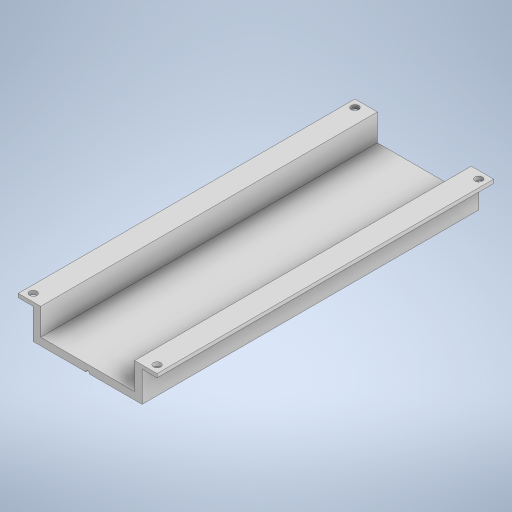
# Autodesk Inventor part: SoporteMaterial
Saved by Autodesk Inventor 2023 (Build 270158000, 158)
## iProperties
Created: 2023-04-09
Part Number: SoporteMaterial
Material: Generic
Document SubType Name: Modeling
Designer: Lenovo
Density: 1 g/cm^3
Appearance: Default
Author: Lenovo
Autodesk Inventor part; units mm, degrees
ref_plane "YZ Plane" through (0, 0, 0) normal (1, 0, 0) x (0, 1, 0)
ref_plane "XZ Plane" through (0, 0, 0) normal (0, 1, 0) x (-1, 0, 0)
ref_plane "XY Plane" through (0, 0, 0) normal (0, 0, 1) x (1, 0, 0)
sketch "Sketch1" plane through (0, 0, 0) normal (0, 0, 1) x (1, 0, 0)
  line L0 (165.5, 18.25) -> (165.5, 13.25)
  line L1 (95.5, -27.5) -> (75.25, -27.5)
  arc A0 (75.25, -27.5) -> (70.25, -27.5) centre (72.75, -27.5) ccw
  line L2 (70.25, -27.5) -> (50, -27.5)
  line L3 (145.5, 0) -> (145.5, 13.25)
  line L4 (145.5, 13.25) -> (165.5, 13.25)
  line L5 (0, 13.25) -> (0, 0)
  line L6 (0, 13.25) -> (-20, 13.25)
  line L7 (-20, 13.25) -> (-20, 18.25)
  line L8 (-20, 18.25) -> (0, 18.25)
  line L9 (0, 18.25) -> (10, 18.25)
  line L10 (10, 18.25) -> (10, -17.5)
  line L11 (165.5, 18.25) -> (145.5, 18.25)
  line L12 (145.5, 18.25) -> (135.5, 18.25)
  line L13 (135.5, 18.25) -> (135.5, -17.5)
  line L14 (135.5, -17.5) -> (10, -17.5)
  line L15 (0, 0) -> (0, -27.5)
  line L16 (0, -27.5) -> (50, -27.5)
  line L17 (95.5, -27.5) -> (145.5, -27.5)
  line L18 (145.5, -27.5) -> (145.5, 0)
  point P0 (0, 0)
  dimension "d0" = 10
  dimension "d1" = 35.75
  dimension "d2" = 10
  constraints: 38 end point, 5 perpendicular, 3 point on line, 2 horizontal, 2 point on circle, 1 centre point, 1 vertical
  measures "d0" distance of L8.end L9.end
  measures "d1" distance of L9.end L10.end
  measures "d2" distance of L11.end L12.end
extrude "Extrusion1" add sketch "Sketch1" along normal blind 450
sketch "Sketch2" plane through (-20, 13.25, 0) normal (0, -1, 0) x (1, 0, 0)
  line L0 (30, 450) -> (0, 450) projected
  line L1 (20, 0) -> (20, 450) projected
  line L2 (0, 450) -> (20, 450)
  line L3 (20, 450) -> (20, 430)
  line L4 (20, 430) -> (0, 430)
  line L5 (0, 430) -> (0, 450)
  circle A0 centre (10, 440) radius 5
  line L6 (185.5, 0) -> (185.5, 450) projected
  line L7 (185.5, 450) -> (165.5, 450)
  line L8 (165.5, 450) -> (165.5, 430)
  line L9 (165.5, 430) -> (185.5, 430)
  line L10 (185.5, 430) -> (185.5, 450)
  line L11 (185.5, 0) -> (155.5, 0) projected
  line L12 (185.5, 0) -> (165.5, 0)
  line L13 (165.5, 0) -> (165.5, 20)
  line L14 (165.5, 20) -> (185.5, 20)
  line L15 (185.5, 20) -> (185.5, 0)
  line L16 (0, 0) -> (0, 450) projected
  line L17 (0, 0) -> (20, 0)
  line L18 (20, 0) -> (20, 20)
  line L19 (20, 20) -> (0, 20)
  line L20 (0, 20) -> (0, 0)
  circle A1 centre (175.5, 440) radius 5
  circle A2 centre (175.5, 10) radius 5
  circle A3 centre (10, 10) radius 5
  dimension "d5" = 20
  dimension "d6" = 10
  dimension "d7" = 20
  dimension "d8" = 20
  dimension "d9" = 20
  dimension "d10" = 20
  dimension "d11" = 20
  dimension "d12" = 20
  dimension "d13" = 10
  dimension "d14" = 10
  dimension "d15" = 10
  constraints: 32 end point, 8 parallel, 4 centre point, 4 horizontal, 4 perpendicular, 1 point on line
  measures "d5" distance of L2.end L3.end
  measures "d6" diameter of A0
  measures "d7" distance of L9.end L8.end
  measures "d8" distance of L8.end L7.end
  measures "d9" distance of L13.end L14.end
  measures "d10" distance of L12.end L13.end
  measures "d11" distance of L19.end L18.end
  measures "d12" distance of L18.end L17.end
  measures "d13" diameter of A1
  measures "d14" diameter of A2
  measures "d15" diameter of A3
extrude "Extrusion2" cut sketch "Sketch2" against normal blind 450 contours A0 | A1 | A2 | A3
body "Solid1"
